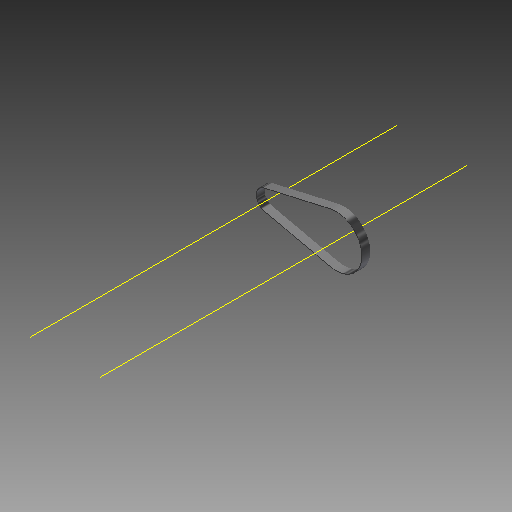
# Autodesk Inventor part: Зубчатый ремень
Saved by Autodesk Inventor 2019.1 (Build 231200000, 200)
## iProperties
Created: 2018-10-15
Part Number: Зубчатый ремень
Material: Rubber
Document SubType Name: Modeling
Designer: Олег
Density: 1 g/cm^3
Appearance: Rubber - Black - Version 1.1
CustomPartVersion: 1
Author: Олег
Autodesk Inventor part; units mm, degrees
sketch "Эскизная траектория" plane through (0, 0, 0) normal (0, 0, 1) x (1, 0, 0)
  arc A0 (-4.509, -19.8692) -> (-4.509, 19.8692) centre (0, 0) ccw
  arc A1 (-57.3198, 7.8846) -> (-57.3198, -7.8846) centre (-55.5305, 0) ccw
  line L0 (-57.3198, 7.8846) -> (-4.509, 19.8692)
  line L1 (-4.509, -19.8692) -> (-57.3198, -7.8846)
  constraints: 4 end point, 4 point on circle, 2 centre point
ref_plane "Плоскость сечения" through (-4.509, 19.8692, 0) normal (-0.9752, -0.2213, 0) x (0, 0, 1)
ref_plane "РабПлоскость2" through (0, 0, 0) normal (-1, 0, 0) x (0, 0, 1)
ref_plane "РабПлоскость3" through (-55.5305, 0, 0) normal (0.9298, -0.3681, 0) x (0, 0, 1)
sketch "Сечение" plane through (-4.509, 19.8692, 0) normal (-0.9752, -0.2213, 0) x (0, 0, 1)
  line L0 (-3.175, 0.381) -> (3.175, 0.381)
  line L1 (3.175, 0.381) -> (3.175, -0.254)
  line L2 (3.175, -0.254) -> (-3.175, -0.254)
  line L3 (-3.175, -0.254) -> (-3.175, 0.381)
  line L4 (-3.175, 0) -> (3.175, 0) construction
  point P0 (0, 0)
  point P1 (0, 0)
  dimension "d0" = 6.35
  dimension "d4" = 0.254
  dimension "d5" = 0.381
  constraints: 10 end point, 2 parallel, 2 point on line, 1 coincident, 1 horizontal, 1 midpoint, 1 perpendicular, 1 other
  measures "d0" distance between parallel lines of L1 L3
  measures "d4" distance between parallel lines of L2 L4
  measures "d5" distance between parallel lines of L4 L0
sweep "Ремень" add profiles "Сечение" path "Эскизная траектория"
equation "\"d0\" = da_B"
equation "\"d4\" = da_a"
equation "\"d5\" = da_a2"
equation "\"da_B\" = 6.35"
equation "\"da_pb\" = 2.032"
equation "\"da_L\" = 203.2"
equation "\"da_a\" = 0.254"
equation "\"da_S\" = 1.143"
equation "\"da_Beta\" = 20deg"
equation "\"da_Ht\" = 0.508"
equation "\"da_H\" = 1.143"
equation "\"da_a2\" = 0.381"
body "Solid1"
